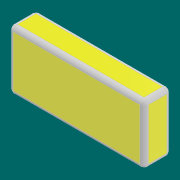
# Autodesk Inventor part: BateriesFinal
Saved by Autodesk Inventor 2020 (Build 240168000, 168)
## iProperties
Created: 2021-02-09
Part Number: BateriesFinal
Material: Generic
Document SubType Name: Modeling
Designer: santi
Density: 1 g/cm^3
Appearance: Default
Author: santi
Autodesk Inventor part; units mm, degrees
ref_plane "YZ Plane" through (0, 0, 0) normal (1, 0, 0) x (0, 1, 0)
ref_plane "XZ Plane" through (0, 0, 0) normal (0, 1, 0) x (-1, 0, 0)
ref_plane "XY Plane" through (0, 0, 0) normal (0, 0, 1) x (1, 0, 0)
sketch "Sketch1" plane through (0, 0, 0) normal (0, 0, 1) x (1, 0, 0)
  line L0 (0, 0) -> (95, 0)
  line L1 (95, 0) -> (95, 42)
  line L2 (95, 42) -> (0, 42)
  line L3 (0, 42) -> (0, 0)
  dimension "d0" = 95
  dimension "d1" = 42
  constraints: 8 end point, 3 perpendicular, 1 horizontal
  measures "d0" distance of L0.start L0.end
  measures "d1" distance of L0.end L1.end
extrude "Extrusion1" add sketch "Sketch1" along normal blind 19
fillet "Fillet1" radius 3 12 edges at (47.5, 42, 19) (47.5, 42, 0) (95, 42, 9.5) (95, 21, 19) (95, 21, 0) (95, 0, 9.5) (47.5, 0, 0) (47.5, 0, 19) (0, 0, 9.5) (0, 21, 19) (0, 21, 0) (0, 42, 9.5)
body "Solid1"
